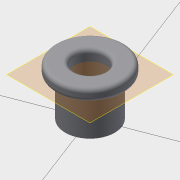
# Autodesk Inventor part: tubeclamp male
Saved by Autodesk Inventor 2014 (Build 180170000, 170)
## iProperties
Created: 2016-05-23
Part Number: tubeclamp male
Material: Generic
Document SubType Name: Modeling
Designer: admin
Density: 1 g/cm^3
Appearance: Default
Author: admin
Autodesk Inventor part; units mm, degrees
ref_plane "YZ Plane" through (0, 0, 0) normal (1, 0, 0) x (0, 1, 0)
ref_plane "XZ Plane" through (0, 0, 0) normal (0, 1, 0) x (-1, 0, 0)
ref_plane "XY Plane" through (0, 0, 0) normal (0, 0, 1) x (1, 0, 0)
ref_plane "Work Plane1" through (0, 0, 0) normal (0, 0, 1) x (1, 0, 0)
sketch "Sketch1" plane through (0, 0, 0) normal (0, 0, 1) x (1, 0, 0)
  circle A0 centre (0, 0) radius 3.25 projected
  circle A1 centre (0, 0) radius 2
  point P0 (0, 0)
  constraints: 1 centre point, 1 coincident
extrude "Extrusion1" add sketch "Sketch1" against normal blind 5
sketch "Sketch2" plane through (0, 0, 0) normal (0, 0, 1) x (1, 0, 0)
  circle A0 centre (0, 0) radius 2 projected
  circle A1 centre (0, 0) radius 3.25 projected
  circle A2 centre (0, 0) radius 4.5
  dimension "d2" = 9
  constraints: 1 centre point, 1 coincident
  measures "d2" diameter of A2
extrude "Extrusion2" add sketch "Sketch2" along normal blind 1.5 contours A1 | A2
fillet "Fillet1" radius 0.5 3 edges at (-4.5, 0, 1.5) (-2, 0, 1.5) (-4.5, 0, 0)
sketch "Sketch3" plane through (0, 0, -5) normal (0, 0, -1) x (-1, 0, 0)
  circle A0 centre (0, 0) radius 2 projected
  circle A1 centre (0, 0) radius 3.25 projected
  circle A2 centre (0, 0) radius 3.55
  dimension "d6" = 0.3
  constraints: 1 centre point, 1 coincident
  measures "d6" radial gap between concentric circles of A1 A2
extrude "Extrusion3" add sketch "Sketch3" along normal mid plane 2 contours A1 | A2
chamfer "Chamfer1" distance 1.5 angle 20 1 edges at (3.55, 0, -6) measured on face at (-3.5385, -0.2857, -4.6667)
fillet "Fillet2" radius 0.5 2 edges at (-3.25, 0, -4) (3.55, 0, -4)
sketch "Sketch4" plane through (0, 0, -6) normal (0, 0, -1) x (-1, 0, 0)
  circle A0 centre (0, 0) radius 3.004 projected
  line L0 (-0.5, 5) -> (0.5, 5)
  line L1 (0.5, 5) -> (0.5, -5)
  line L2 (0.5, -5) -> (-0.5, -5)
  line L3 (-0.5, -5) -> (-0.5, 5)
  line L4 (-0.5, 5) -> (0.5, -5) construction
  line L5 (0.5, 5) -> (-0.5, -5) construction
  line L6 (-6, 0.5) -> (6, 0.5)
  line L7 (6, 0.5) -> (6, -0.5)
  line L8 (6, -0.5) -> (-6, -0.5)
  line L9 (-6, -0.5) -> (-6, 0.5)
  line L10 (-6, 0.5) -> (6, -0.5) construction
  line L11 (6, 0.5) -> (-6, -0.5) construction
  dimension "d13" = 1
  dimension "d14" = 10
  dimension "d15" = 1
  constraints: 24 end point, 4 midpoint, 4 parallel, 2 horizontal, 2 perpendicular
  measures "d13" distance of L1.end L2.end
  measures "d14" distance of L0.end L1.end
  measures "d15" distance of L6.end L7.end
extrude "Extrusion4" cut sketch "Sketch4" against normal blind 5 contours A0 L8 L1 L6 | A0 L6 L7 L8 | L1 L6 L3 A0 | A0 L3 L0 L1 | L1 L8 L3 L6 | L1 L2 L3 A0 | A0 L3 L8 L1 | L3 L8 A0 L6 | A0 L8 L9 L6
body "Solid1"
